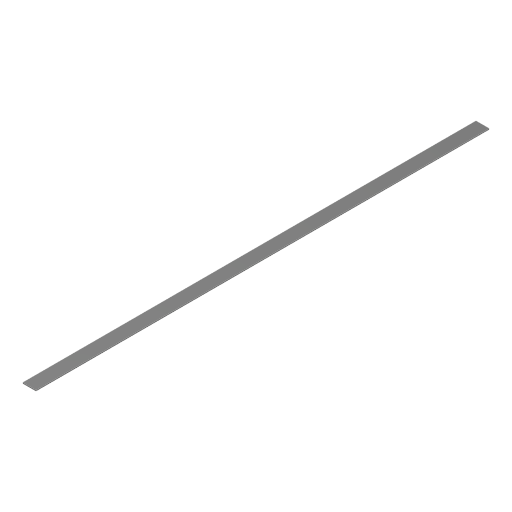
# Autodesk Inventor part: MTAZ-500-50-1
Saved by Autodesk Inventor 2024.3 (Build 283343000, 343)
## iProperties
Created: 2025-06-09
Part Number: MTAZ-500-50-1
Material: Generic
Document SubType Name: Modeling
Designer: MPA
Density: 1 g/cm^3
Appearance: Smooth - Black
Author: MPA
Autodesk Inventor part; units mm, degrees
ref_plane "YZ Plane" through (0, 0, 0) normal (1, 0, 0) x (0, 1, 0)
ref_plane "XZ Plane" through (0, 0, 0) normal (0, 1, 0) x (-1, 0, 0)
ref_plane "XY Plane" through (0, 0, 0) normal (0, 0, 1) x (1, 0, 0)
sketch "Sketch1" plane through (0, 0, 0) normal (0, 1, 0) x (-1, 0, 0)
  line L0 (-10, 340) -> (10, 340)
  line L1 (10, 340) -> (10, -340)
  line L2 (10, -340) -> (-10, -340)
  line L3 (-10, -340) -> (-10, 340)
  line L4 (-10, 340) -> (10, -340) construction
  line L5 (10, 340) -> (-10, -340) construction
  point P0 (0, 0)
  dimension "d0" = 20
  dimension "d1" = 680
  constraints: 12 end point, 2 midpoint, 2 parallel, 1 horizontal, 1 perpendicular
  measures "d0" distance of L1.end L2.end
  measures "d1" distance of L0.end L1.end
extrude "Extrusion1" add sketch "Sketch1" along normal blind 1.4
body "Solid1"
